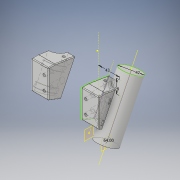
# Autodesk Inventor part: DNM-USD8-Fix
Saved by Autodesk Inventor 2019.3 (Build 233278000, 278)
## iProperties
Created: 2019-01-16
Part Number: DNM-USD8-Fix
Material: Generic
Document SubType Name: Modeling
Designer: eroldan
Density: 1 g/cm^3
Appearance: Default
Author: eroldan
Autodesk Inventor part; units mm, degrees
ref_plane "XZ Plane" through (0, 0, 0) normal (0, 1, 0) x (-1, 0, 0)
ref_plane "Work Plane2" through (69.75, 0, 0) normal (1, 0, 0) x (0, 1, 0)
sketch "Sketch2" plane through (69.75, 0, 0) normal (1, 0, 0) x (0, 1, 0)
  line L0 (0, 0) -> (0, 9.6252) construction
  line L1 (0, 0) -> (104.9991, -51.2115)
  dimension "headtube_angle" = 64
  constraints: 4 end point, 1 vertical
  measures "headtube_angle" angle of L0 L1
ref_plane "Work Plane3" through (69.75, 104.9991, -51.2115) normal (0, 0.898794, -0.4383711) x (-1, 0, 0)
sketch "Sketch3" plane through (69.75, 104.9991, -51.2115) normal (0, 0.898794, -0.4383711) x (-1, 0, 0)
  circle A0 centre (0, 0) radius 21
  point P0 (69.75, 0)
  dimension "diameter_stanchions" = 42
  constraints: 1 centre point
  measures "diameter_stanchions" diameter of A0
sweep "Sweep1" add profiles "Sketch3" path "Sketch2"
ref_plane "Work Plane4" through (34.25, 0, 0) normal (1, 0, 0) x (0, 1, 0)
sketch "Sketch4" plane through (34.25, 0, 0) normal (1, 0, 0) x (0, 1, 0)
  line L0 (0, 0) -> (104.9991, -51.2115) construction
  line L1 (83.3693, -40.6619) -> (21.2622, -10.3703)
  line L2 (21.2622, -10.3703) -> (31.9009, 15.5814)
  line L3 (31.9009, 15.5814) -> (90.0087, 15.5814)
  line L4 (90.0087, 1.6677) -> (83.3693, -40.6619)
  line L5 (83.3693, -40.6619) -> (90.0087, 1.6677)
  line L6 (90.0087, 15.5814) -> (90.0087, 1.6677)
  constraints: 12 end point, 2 point on line, 1 vertical
extrude "Extrusion1" add sketch "Sketch4" along normal up to surface (35.5 mm away) separate body
ref_plane "Work Plane5" through (34.25, 31.9009, -53.6686) normal (0, 0, 1) x (1, 0, 0)
sketch "Sketch6" plane through (34.25, 31.9009, -53.6686) normal (0, 0, 1) x (1, 0, 0)
  line L0 (-34.25, 106.9862) -> (-34.25, -65.7888) construction
  point P0 (-34.25, -31.9009)
  point P1 (8.75, 41.0717)
  point P2 (8.75, 13.0717)
  dimension "d11" = 28
  dimension "distance_lamp_holes" = 43
  constraints: 1 vertical alignment
  measures "d11" distance of point (8.75, 13.072) point (8.75, 41.072)
  measures "distance_lamp_holes" distance from line of L0 point (8.75, 41.072)
hole "Hole1" at (43, 72.9726, -53.6686) at (43, 44.9726, -53.6686) direction (0, 0, 1) diameter 5.5 end through all counterbore diameter 9.3 counterbore depth 54.75 bodies 2
combine bodies "Combine1" operation type subtract main body 2 bodies to subtract 1 keep tools yes
sketch "Sketch9" plane through (69.75, 31.9009, 15.5814) normal (1, 0, 0) x (0, 0, -1)
  line L0 (-3.2933, -22.6951) -> (47.9182, 82.304) construction
  line L1 (21.898, 34.6577) -> (25.6242, 42.2975)
  line L2 (25.6242, 42.2975) -> (23.1975, 43.4811)
  line L3 (23.1975, 43.4811) -> (19.4713, 35.8413)
  line L4 (19.4713, 35.8413) -> (21.898, 34.6577)
  line L5 (10.5049, 11.2983) -> (6.7787, 3.6585)
  line L6 (6.7787, 3.6585) -> (4.352, 4.8421)
  line L7 (4.352, 4.8421) -> (8.0781, 12.4819)
  line L8 (8.0781, 12.4819) -> (10.5049, 11.2983)
  line L9 (-4.8169, -73.7235) -> (87.1911, 114.9209) projected
  point P0 (15.5814, -31.9009)
  dimension "d27" = 8.5
  dimension "d28" = 2.7
  dimension "d29" = 2.5
  dimension "d30" = 8.5
  dimension "d33" = 2.5
  dimension "d34" = 2.7
  constraints: 16 end point, 5 perpendicular, 1 parallel
  measures "d27" distance of L1.start L1.end
  measures "d28" distance of L1.end L2.end
  measures "d29" distance between parallel lines of L0 L1
  measures "d30" distance of L5.start L5.end
  measures "d33" distance between parallel lines of L0 L5
  measures "d34" distance of L7.end L5.start
revolve "Revolution1" cut sketch "Sketch9" angle 360 about axis through (69.75, 0, 0) along (0, 0.898794, -0.4383711) bodies 2
fillet "Fillet3" radius 1.5 13 edges at (52, 90.0087, 15.5814) (69.75, 60.9548, 15.5814) (69.75, 90.0087, 8.6245) (52, 31.9009, 15.5814) (34.25, 60.9548, 15.5814) (34.25, 86.689, -19.4971) (34.25, 90.0087, 8.6245) (52, 90.0087, 1.6677) (69.75, 88.3912, -8.645) (41.5, 83.3693, -40.6619) (34.25, 26.5816, 2.6056) (41.5, 21.2622, -10.3703) (34.25, 52.3158, -25.5161)
sketch "Sketch10" plane through (35.75, 89.9906, 1.5522) normal (0, 0.9879214, -0.1549558) x (1, 0, 0)
  line L0 (0, 40.6999) -> (13.0899, 40.6999) projected
  line L1 (11.9, 39.3317) -> (11.9, 3.1021) construction
  line L2 (2.6, 39.3317) -> (2.6, 3.1021) construction
  line L3 (11.9, 39.3317) -> (11.9, 3.1021) construction
  line L4 (11.9, 23.526) -> (2.6, 23.526) construction
  point P0 (-35.75, 15.478)
  point P1 (7.25, 26.6999)
  point P2 (7.25, 23.526)
  dimension "d35" = 14
  constraints: 2 end point, 2 point on line, 1 midpoint, 1 perpendicular, 1 vertical alignment
  measures "d35" distance from line of point (7.25, 26.7) L0
hole "Hole2" at (43, 85.8533, -24.8252) direction (0, -0.9879214, 0.1549558) diameter 5.25 end up to surface bodies 2
mirror "Mirror3" about plane through (0, 0, 0) normal (1, 0, 0) bodies 2
equation "\"d30\" = d27"
equation "\"d33\" = d29"
equation "\"d34\" = d28"
